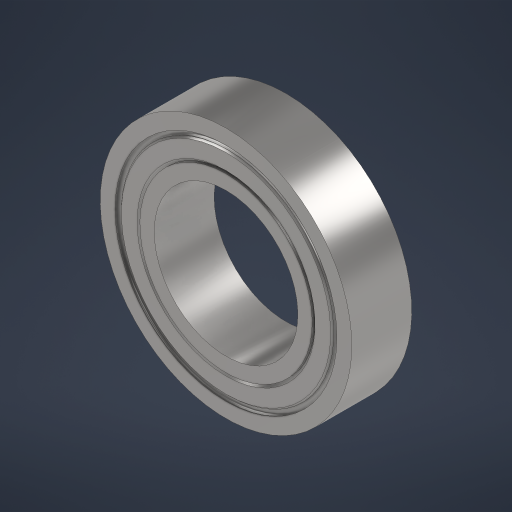
# Autodesk Inventor part: wheel bearing
Saved by Autodesk Inventor 2023 (Build 270158000, 158)
## iProperties
Created: 2023-03-15
Part Number: wheel bearing
Material: Типовые
Document SubType Name: Modeling
Designer: Khasal
Density: 5.2264 g/cm^3
Appearance: С умеренной полировкой
Mass: 6 g
Surface Area: 10.7074 cm^2
Volume: 1.14802 cm^3
Author: Khasal
Autodesk Inventor part; units mm, degrees
ref_plane "YZ Plane" through (0, 0, 0) normal (1, 0, 0) x (0, 1, 0)
ref_plane "XZ Plane" through (0, 0, 0) normal (0, 1, 0) x (-1, 0, 0)
ref_plane "XY Plane" through (0, 0, 0) normal (0, 0, 1) x (1, 0, 0)
sketch "Эскиз1" plane through (0, 0, 0) normal (1, 0, 0) x (0, 1, 0)
  line L0 (6, -2.5) -> (6, 2.5)
  line L1 (10.5, 2.5) -> (10.5, -2.5)
  arc A0 (8.8667, 2.3707) -> (9.2616, 2.5) centre (9.0853, 2.3707) ccw
  line L2 (8.8667, 2.3707) -> (8.7374, 2.5)
  line L3 (8.8667, 2.3707) -> (9.0495, 2.3707) construction
  line L4 (7.4323, 2.5) -> (7.196, 2.2638)
  line L5 (7.4323, 2.5) -> (7.8016, 2.5) construction
  line L6 (9.2616, 2.5) -> (10.5, 2.5)
  line L7 (6, 2.5) -> (7.196, 2.5)
  line L8 (7.4323, 2.5) -> (8.7374, 2.5)
  line L9 (7.196, 2.5) -> (7.196, 2.2638)
  line L10 (9.696, 0) -> (8.6749, 0)
  arc A1 (9.2616, -2.5) -> (8.8667, -2.3707) centre (9.0853, -2.3707) ccw
  line L11 (8.8667, -2.3707) -> (8.7374, -2.5)
  line L12 (8.8667, -2.3707) -> (9.0495, -2.3707) construction
  line L13 (7.4323, -2.5) -> (7.196, -2.2638)
  line L14 (7.4323, -2.5) -> (7.8016, -2.5) construction
  line L15 (9.2616, -2.5) -> (10.5, -2.5)
  line L16 (6, -2.5) -> (7.196, -2.5)
  line L17 (7.4323, -2.5) -> (8.7374, -2.5)
  line L18 (7.196, -2.5) -> (7.196, -2.2638)
  line L19 (10.5, -2.5) -> (9.2616, -2.5)
  line L20 (8.7374, -2.5) -> (7.4323, -2.5)
  line L21 (7.196, -2.5) -> (6, -2.5)
  line L22 (0, -3.5047) -> (0, 3.5047) projected
  point P0 (0, 0)
  point P1 (9.304, 2.5)
  point P2 (9.304, -2.5)
  dimension "d0" = 5
  dimension "d1" = 4.5
  dimension "d2" = 6
  dimension "d5" = 135
  dimension "d6" = 135
  constraints: 44 end point, 10 parallel, 10 symmetric about line, 6 horizontal, 4 point on circle, 3 perpendicular, 2 centre point, 2 point on line, 1 equal length, 1 other
  measures "d0" distance of L0.start L0.end
  measures "d1" distance of L1.end L0.start
  measures "d2" distance from line of L0 point (0, 0)
  measures "d5" angle of L3 L2
  measures "d6" angle of L4 L5
revolve "Вращение1" add sketch "Эскиз1" angle 360 about axis through (0, 0, -10) along (0, 0, 1)
